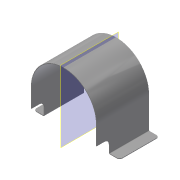
# Autodesk Inventor part: Guard, Shaft
Saved by Autodesk Inventor 2021 (Build 250183000, 183)
## iProperties
Created: 2013-05-06
Part Number: Guard, Shaft
Material: Steel, Mild
Document SubType Name: Sheet Metal
Designer: user
Mass: 5217.42 g
Surface Area: 4423.68 cm^2
Volume: 663.794 cm^3
Density: 7.86 g/cm^3
Sheet Metal Rule: Default
Appearance: Steel
Author: user
Autodesk Inventor part; units mm, degrees
ref_plane "YZ Plane" through (0, 0, 0) normal (1, 0, 0) x (0, 1, 0)
ref_plane "XZ Plane" through (0, 0, 0) normal (0, 1, 0) x (-1, 0, 0)
ref_plane "XY Plane" through (0, 0, 0) normal (0, 0, 1) x (1, 0, 0)
sketch "Sketch1" plane through (0, 0, 0) normal (0, 0, 1) x (1, 0, 0)
  line L0 (-152.4, -152.4) -> (-152.4, 0)
  arc A0 (152.4, 0) -> (-152.4, 0) centre (0, 0) ccw
  line L1 (152.4, 0) -> (152.4, -152.4)
  dimension "d0" = 152.4
  dimension "d2" = 304.8
  measures "d0" distance of L0.start L0.end
  measures "d2" distance between parallel lines of L1 L0
contour flange "Contour Flange1" sketch "Sketch1" thickness 3.048 bend radius 3.048 width 247.65 along (0, 0, 1) mid plane no both sides no wall seen from (152.4, -76.2, 0) lies toward (1, 0, 0) curves L1 A0 L0
bend "Bend1"
corner "Corner1"
ref_plane "Work Plane1" through (-1.524, 0, 0) normal (-1, 0, 0) x (0, 0, 1)
sketch "Sketch2" plane through (-152.4, -149.352, 247.65) normal (0, -1, 0) x (1, 0, 0)
  line L0 (0, -247.65) -> (0, 0)
  line L1 (0, 0) -> (-50.8, 0)
  line L2 (-50.8, 0) -> (-50.8, -247.65)
  line L3 (-50.8, -247.65) -> (0, -247.65)
  constraints: 4 end point, 4 other
edge flange "Flange1" height 50.8 angle 90 thickness 3.048 bend radius 3.048 thickness toward (0, -1, 0) relief straight relief width 3.048 relief depth 1.524 corner gap 3.048 corner form 0 edges at (-155.448, -152.4, 123.825) (155.448, -152.4, 123.825) wall of the first edge with corners at (-152.4, -149.352, 0) (-152.4, -149.352, 247.65) (-203.2, -149.352, 247.65) (-203.2, -149.352, 0)
bend "Bend2"
corner "Corner2"
sketch "Sketch3" plane through (-1.524, 0, 0) normal (-1, 0, 0) x (0, 0, 1)
  line L0 (0, -146.304) -> (247.65, -146.304)
  line L1 (247.65, -146.304) -> (247.65, 0)
  line L2 (0, 0) -> (247.65, 0)
  line L3 (0, -146.304) -> (0, 0)
  line L4 (288.2554, -179.7405) -> (186.8167, -179.7405)
  line L5 (186.8167, -179.7405) -> (186.8167, -89.6359)
  line L6 (186.8167, -89.6359) -> (288.2554, -89.6359)
  line L7 (288.2554, -89.6359) -> (288.2554, -179.7405)
  point P0 (247.65, 0)
  constraints: 16 end point, 2 parallel, 1 horizontal, 1 perpendicular
extrude "Extrusion1" cut sketch "Sketch3" along normal through all both and the other way through all contours L5 L6 L1 L0 | L0 L1 L6 L7 L4 L5
fillet "Corner Round2" radius 25.4 2 edges at (-153.924, -89.6359, 186.8167) (153.924, -89.6359, 186.8167)
fillet "Corner Round1" radius 12.7 4 edges at (-203.2, -150.876, 0) (203.2, -150.876, 0) (-203.2, -150.876, 186.8167) (203.2, -150.876, 186.8167)
equation "\"d3\" = BendReliefWidth"
equation "\"d4\" = BendReliefDepth"
equation "\"d5\" = MinimumRemnant"
equation "\"d6\" = BendRadius"
equation "\"d8\" = BendRadius"
equation "\"d10\" = CornerReliefSize"
equation "\"d11\" = GapSize"
equation "\"d12\" = JacobiRadiusSize"
equation "\"d27\" = Thickness"
equation "\"d13\" = BendReliefWidth"
equation "\"d14\" = BendReliefDepth"
equation "\"d15\" = MinimumRemnant"
equation "\"d16\" = BendRadius"
equation "\"d19\" = BendRadius"
equation "\"d20\" = CornerReliefSize"
equation "\"d21\" = GapSize"
equation "\"d22\" = JacobiRadiusSize"
equation "\"BendRadius\" = Thickness"
equation "\"BendReliefWidth\" = Thickness"
equation "\"BendReliefDepth\" = 0.5 * Thickness"
equation "\"CornerReliefSize\" = 4 * Thickness"
equation "\"MinimumRemnant\" = 2 * Thickness"
equation "\"TransitionRadius\" = BendRadius"
equation "\"JacobiRadiusSize\" = Thickness"
equation "\"GapSize\" = Thickness"
equation "\"Thickness\" = 3.048"
body "Solid1"
